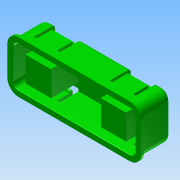
# Autodesk Inventor part: Two Block Socket
Saved by Autodesk Inventor 2015 (Build 190159000, 159)
## iProperties
Created: 2012-02-21
Part Number: Two Block Socket
Material: Generic
Document SubType Name: Modeling
Designer: Thom Tremblay
Density: 1 g/cm^3
Appearance: Dark Green
Author: Thom Tremblay
Autodesk Inventor part; units mm, degrees
ref_plane "XY Plane" through (0, 0, 0) normal (0, 0, 1) x (1, 0, 0)
sketch "Sketch1" plane through (0, 0, 0) normal (0, 0, 1) x (1, 0, 0)
  line L0 (0, 0) -> (30.48, 0)
  line L1 (30.48, 0) -> (30.48, 11.811)
  line L2 (30.48, 11.811) -> (0, 11.811)
  line L3 (0, 11.811) -> (0, 0)
  dimension "d0" = 30.48
  dimension "d1" = 11.811
  constraints: 8 end point, 2 parallel, 1 horizontal, 1 perpendicular
  measures "d0" distance of L2.end L1.end
  measures "d1" distance of L1.end L0.end
extrude "Extrusion1" add sketch "Sketch1" along normal blind 14.478
fillet "Fillet1" radius 5.08 1 edges at (30.48, 11.811, 7.239)
shell "Shell1" thickness 2.54 removed faces 3 at (0, 7.874, 4.826) at (18.6267, 3.937, 14.478) at (10.16, 0, 4.826) ; own thickness 1.27 on faces at (18.6267, 3.937, 0)
sketch "Sketch2" plane through (0, 0, 1.27) normal (0, 0, 1) x (1, 0, 0)
  line L0 (27.94, 0) -> (0, 0) construction
  line L1 (11.303, 0) -> (22.987, 0)
  line L2 (22.987, 0) -> (22.987, 5.7977)
  line L3 (22.987, 5.7977) -> (11.303, 5.7977)
  line L4 (11.303, 5.7977) -> (11.303, 0)
  dimension "d7" = 11.684
  dimension "d8" = 5.7977
  dimension "d26" = 11.303
  constraints: 8 end point, 2 parallel, 1 horizontal, 1 perpendicular, 1 point on line
  measures "d7" distance of L1.start L1.end
  measures "d8" distance of L1.end L2.end
  measures "d26" distance from line of L0.end L4
ref_plane "Work Plane1" through (0, 0, 13.6398) normal (0, 0, 1) x (1, 0, 0)
sketch "Sketch3" plane through (0, 11.811, 14.478) normal (0, 1, 0) x (1, 0, 0)
  line L0 (25.4, 14.478) -> (0, 14.478) projected
  line L1 (23.241, 14.478) -> (11.303, 14.478)
  line L2 (11.303, 14.478) -> (11.303, 4.7675)
  line L3 (11.303, 4.7675) -> (23.241, 4.7675)
  line L4 (23.241, 4.7675) -> (23.241, 14.478)
  line L5 (12.573, 4.7675) -> (21.971, 4.7675)
  line L6 (21.971, 4.7675) -> (21.971, 11.938)
  line L7 (21.971, 11.938) -> (12.573, 11.938)
  line L8 (12.573, 11.938) -> (12.573, 4.7675)
  line L9 (21.971, 11.938) -> (12.573, 11.938)
  line L10 (12.573, 11.938) -> (12.573, 10.668)
  line L11 (12.573, 10.668) -> (21.971, 10.668)
  line L12 (21.971, 10.668) -> (21.971, 11.938)
  line L13 (0, 14.478) -> (0, 0) projected
  point P0 (17.272, 4.7675)
  dimension "d14" = 11.938
  dimension "d15" = 1.27
  dimension "d16" = 2.54
  dimension "d17" = 1.27
  dimension "d27" = 11.303
  constraints: 24 end point, 6 parallel, 3 horizontal, 3 perpendicular, 2 midpoint, 2 point on line
  measures "d14" distance of L2.end L3.end
  measures "d15" distance between parallel lines of L2 L8
  measures "d16" distance between parallel lines of L0 L7
  measures "d17" distance between parallel lines of L11 L7
  measures "d27" distance between parallel lines of L13 L2
shell "Shell2" thickness 1.27 removed faces 6 at (16.9333, 11.811, 4.826) at (27.2559, 11.4598, 4.826) at (30.48, 2.2437, 4.826) at (18.6267, 3.937, 0) at (0, 10.9643, 5.2493) at (19.4733, 0, 0.4233)
extrude "Extrusion3" cut sketch "Sketch3" against normal blind 3.81 contours L4 L3 L6 L7 L8 L2 L0
ref_plane "Work Plane2" through (0, 8.509, 14.478) normal (0, -1, 0) x (1, 0, 0)
extrude "Extrusion4" add sketch "Sketch3" against normal up to surface (2.032 mm away) from surface at -1.27 contours L11 L8 L7 L6
full round fillet "Fillet6" first side at (15.7057, 9.017, 3.81) centre faces at (18.8383, 8.509, 2.9633) second side at (18.8383, 9.8637, 2.54)
full round fillet "Fillet3" first side at (23.241, 10.1177, 3.6602) centre faces at (22.3943, 10.1177, 9.7105) second side at (21.971, 10.1177, 5.3535)
full round fillet "Fillet4" first side at (11.303, 10.1177, 3.6602) centre faces at (11.7263, 10.1177, 9.7105) second side at (12.573, 10.1177, 5.3535)
extrude "Extrusion2" add sketch "Sketch2" along normal up to surface (12.3698 mm away)
fillet "Fillet2" radius 0.127 9 edges at (27.1961, 8.5271, 1.27) (27.94, 3.3655, 1.27) (5.6515, 9.271, 1.27) (24.3205, 9.271, 1.27) (11.303, 5.7977, 7.4549) (17.145, 5.7977, 13.6398) (22.987, 5.7977, 7.4549) (22.987, 2.8988, 13.6398) (11.303, 2.8988, 13.6398)
fillet "Fillet2" radius 0.254 3 edges at (27.1961, 8.5271, 14.478) (27.94, 3.3655, 14.478) (12.7, 9.271, 14.478)
fillet "Fillet7" radius 1.27 4 edges at (29.21, 3.3655, 0) (24.3205, 10.541, 0) (28.0941, 9.4251, 0) (5.6515, 10.541, 0)
mirror "Mirror1" about plane through (0, 0, 0) normal (-1, 0, 0)
mirror "Mirror2" about plane through (30.48, 0, 0) normal (0, -1, 0)
body "Solid1"
